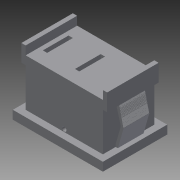
# Autodesk Inventor part: Base
Saved by Autodesk Inventor 2015 (Build 190159000, 159)
## iProperties
Created: 2016-05-14
Part Number: Base
Material: Genérico
Document SubType Name: Modeling
Designer: Isra
Density: 1 g/cm^3
Appearance: Valor por defecto
Author: Isra
Autodesk Inventor part; units mm, degrees
ref_plane "YZ Plane" through (0, 0, 0) normal (1, 0, 0) x (0, 1, 0)
ref_plane "XZ Plane" through (0, 0, 0) normal (0, 1, 0) x (-1, 0, 0)
ref_plane "XY Plane" through (0, 0, 0) normal (0, 0, 1) x (1, 0, 0)
sketch "Boceto1" plane through (0, 0, 0) normal (0, 0, 1) x (1, 0, 0)
  line L0 (10.5, -7.5) -> (-10.5, -7.5)
  line L1 (-10.5, -7.5) -> (-10.5, 7.5)
  line L2 (-10.5, 7.5) -> (10.5, 7.5)
  line L3 (10.5, 7.5) -> (10.5, -7.5)
  line L4 (10.5, -7.5) -> (-10.5, 7.5) construction
  line L5 (-10.5, -7.5) -> (10.5, 7.5) construction
  point P0 (0, 0)
  dimension "d0" = 21
  dimension "d1" = 15
  constraints: 12 end point, 2 midpoint, 2 parallel, 1 horizontal, 1 perpendicular
  measures "d0" distance of L1.end L2.end
  measures "d1" distance of L0.end L1.end
extrude "Extrusión1" add sketch "Boceto1" along normal blind 2
sketch "Boceto2" plane through (0, 0, 2) normal (0, 0, 1) x (1, 0, 0)
  line L0 (9, -6) -> (-9, -6)
  line L1 (-9, -6) -> (-9, 6)
  line L2 (-9, 6) -> (9, 6)
  line L3 (9, 6) -> (9, -6)
  line L4 (9, -6) -> (-9, 6) construction
  line L5 (-9, -6) -> (9, 6) construction
  point P0 (0, 0)
  dimension "d4" = 18
  dimension "d5" = 12
  constraints: 12 end point, 2 midpoint, 2 parallel, 1 horizontal, 1 perpendicular
  measures "d4" distance of L1.end L2.end
  measures "d5" distance of L0.end L1.end
extrude "Extrusión2" add sketch "Boceto2" along normal blind 11
sketch "Boceto3" plane through (-9, -6, 2) normal (0, -1, 0) x (1, 0, 0)
  line L0 (18, 11) -> (18, 13)
  line L1 (18, 13) -> (19, 13)
  line L2 (19, 13) -> (19, 9)
  line L3 (19, 9) -> (18, 9)
  line L4 (18, 0) -> (18, 11) projected
  line L5 (18, 9) -> (18, 11)
  point P0 (9, -2)
  dimension "d8" = 2
  dimension "d9" = 1
  dimension "d10" = 4
  dimension "d11" = 1
  constraints: 10 end point, 2 perpendicular, 1 collinear, 1 point on line, 1 vertical
  measures "d8" distance of L0.start L0.end
  measures "d9" distance of L0.end L1.end
  measures "d10" distance of L1.end L2.end
  measures "d11" distance of L2.end L3.end
extrude "Extrusión3" add sketch "Boceto3" against normal blind 12
ref_plane "Plano de trabajo1" through (0, -6, 2) normal (1, 0, 0) x (0, 0, -1)
mirror "Simetría1" about plane through (0, -6, 2) normal (1, 0, 0) of "Extrusión3"
sketch "Boceto4" plane through (0, -6, 2) normal (-1, 0, 0) x (0, 0, -1)
  point P0 (2, 6)
ref_plane "Plano de trabajo3" through (-9, 0, 2) normal (0, -1, 0) x (1, 0, 0)
sketch "Boceto5" plane through (-9, 0, 2) normal (0, -1, 0) x (1, 0, 0)
  line L0 (18, 0) -> (18, 9) projected
  line L1 (18, 9) -> (19, 9) projected
  line L2 (19, 9) -> (18, 9) projected
  line L3 (0, 0) -> (18, 0) projected
  line L4 (18, 0) -> (0, 0) projected
  line L5 (-1.5, 0) -> (19.5, 0) projected
  line L6 (19.5, 0) -> (-1.5, 0) projected
  line L7 (18.7905, 9) -> (19.8289, 4.7159)
  line L8 (19.8289, 4.7159) -> (18.5, 0)
  line L9 (-1.5, 0) -> (19.5, 0) projected
  line L10 (18.5, 0) -> (18, 0)
  line L11 (18.7905, 9) -> (18, 9)
  point P0 (9, -2)
  constraints: 8 end point, 1 collinear, 1 horizontal, 1 point on line, 2 other
extrude "Extrusión4" add sketch "Boceto5" along normal blind 3 separate body
sketch "Boceto6" plane through (-9, 0, 2) normal (0, 1, 0) x (1, 0, 0)
  line L0 (18, -9) -> (18, 0) projected
  line L1 (18, 0) -> (18, -9) projected
  line L2 (18, -0.6327) -> (19.1944, -4.78)
  line L3 (19.1944, -4.78) -> (18, -9)
  line L4 (18, -9) -> (18, -0.6327)
  point P0 (9, 2)
  constraints: 6 end point, 1 collinear, 1 point on line
extrude "Extrusión5" cut sketch "Boceto6" against normal blind 3 bodies 2
sketch "Boceto8" plane through (-9, 0, 2) normal (0, 1, 0) x (1, 0, 0)
  line L0 (19.9491, -4.6303) -> (19.748, -4.8063)
  line L1 (19.748, -4.8063) -> (19.874, -4.9502)
  line L2 (19.874, -4.9502) -> (20.0751, -4.7743)
  line L3 (20.0751, -4.7743) -> (19.9491, -4.6303)
  line L4 (19.9169, -4.752) -> (19.7158, -4.928)
  line L5 (19.7158, -4.928) -> (19.8418, -5.072)
  line L6 (19.8418, -5.072) -> (20.0429, -4.896)
  line L7 (20.0429, -4.896) -> (19.9169, -4.752)
  line L8 (19.8931, -4.857) -> (19.692, -5.033)
  line L9 (19.692, -5.033) -> (19.818, -5.1769)
  line L10 (19.818, -5.1769) -> (20.0191, -5.0009)
  line L11 (20.0191, -5.0009) -> (19.8931, -4.857)
  line L12 (19.8635, -4.9773) -> (19.6624, -5.1533)
  line L13 (19.6624, -5.1533) -> (19.7883, -5.2972)
  line L14 (19.7883, -5.2972) -> (19.9895, -5.1212)
  line L15 (19.9895, -5.1212) -> (19.8635, -4.9773)
  line L16 (19.8344, -5.0996) -> (19.6333, -5.2756)
  line L17 (19.6333, -5.2756) -> (19.7593, -5.4196)
  line L18 (19.7593, -5.4196) -> (19.9604, -5.2436)
  line L19 (19.9604, -5.2436) -> (19.8344, -5.0996)
  line L20 (19.8044, -5.2221) -> (19.6033, -5.3981)
  line L21 (19.6033, -5.3981) -> (19.7293, -5.5421)
  line L22 (19.7293, -5.5421) -> (19.9304, -5.3661)
  line L23 (19.9304, -5.3661) -> (19.8044, -5.2221)
  line L24 (19.7757, -5.3446) -> (19.5745, -5.5206)
  line L25 (19.5745, -5.5206) -> (19.7005, -5.6646)
  line L26 (19.7005, -5.6646) -> (19.9016, -5.4886)
  line L27 (19.9016, -5.4886) -> (19.7757, -5.3446)
  line L28 (19.7457, -5.4697) -> (19.5445, -5.6456)
  line L29 (19.5445, -5.6456) -> (19.6705, -5.7896)
  line L30 (19.6705, -5.7896) -> (19.8716, -5.6136)
  line L31 (19.8716, -5.6136) -> (19.7457, -5.4697)
  line L32 (19.7144, -5.5909) -> (19.5133, -5.7669)
  line L33 (19.5133, -5.7669) -> (19.6392, -5.9109)
  line L34 (19.6392, -5.9109) -> (19.8404, -5.7349)
  line L35 (19.8404, -5.7349) -> (19.7144, -5.5909)
  line L36 (19.6844, -5.7159) -> (19.4833, -5.8919)
  line L37 (19.4833, -5.8919) -> (19.6092, -6.0359)
  line L38 (19.6092, -6.0359) -> (19.8104, -5.8599)
  line L39 (19.8104, -5.8599) -> (19.6844, -5.7159)
  line L40 (19.6557, -5.8384) -> (19.4545, -6.0144)
  line L41 (19.4545, -6.0144) -> (19.5805, -6.1584)
  line L42 (19.5805, -6.1584) -> (19.7816, -5.9824)
  line L43 (19.7816, -5.9824) -> (19.6557, -5.8384)
  line L44 (19.6257, -5.9609) -> (19.4245, -6.1369)
  line L45 (19.4245, -6.1369) -> (19.5505, -6.2809)
  line L46 (19.5505, -6.2809) -> (19.7516, -6.1049)
  line L47 (19.7516, -6.1049) -> (19.6257, -5.9609)
  line L48 (19.5969, -6.0797) -> (19.3958, -6.2557)
  line L49 (19.3958, -6.2557) -> (19.5217, -6.3996)
  line L50 (19.5217, -6.3996) -> (19.7229, -6.2236)
  line L51 (19.7229, -6.2236) -> (19.5969, -6.0797)
  line L52 (19.5669, -6.1997) -> (19.3658, -6.3757)
  line L53 (19.3658, -6.3757) -> (19.4917, -6.5196)
  line L54 (19.4917, -6.5196) -> (19.6929, -6.3437)
  line L55 (19.6929, -6.3437) -> (19.5669, -6.1997)
  line L56 (19.5369, -6.3235) -> (19.3358, -6.4994)
  line L57 (19.3358, -6.4994) -> (19.4617, -6.6434)
  line L58 (19.4617, -6.6434) -> (19.6629, -6.4674)
  line L59 (19.6629, -6.4674) -> (19.5369, -6.3235)
  line L60 (19.5202, -6.4655) -> (19.3191, -6.6415)
  line L61 (19.3191, -6.6415) -> (19.4451, -6.7855)
  line L62 (19.4451, -6.7855) -> (19.6462, -6.6095)
  line L63 (19.6462, -6.6095) -> (19.5202, -6.4655)
  line L64 (19.488, -6.5873) -> (19.2869, -6.7632)
  line L65 (19.614, -6.7312) -> (19.488, -6.5873)
  line L66 (19.2869, -6.7632) -> (19.4129, -6.9072)
  line L67 (19.4129, -6.9072) -> (19.614, -6.7312)
  line L68 (19.4643, -6.6922) -> (19.2631, -6.8682)
  line L69 (19.5902, -6.8362) -> (19.4643, -6.6922)
  line L70 (19.2631, -6.8682) -> (19.3891, -7.0121)
  line L71 (19.3891, -7.0121) -> (19.5902, -6.8362)
  line L72 (19.4346, -6.8125) -> (19.2335, -6.9885)
  line L73 (19.5606, -6.9565) -> (19.4346, -6.8125)
  line L74 (19.2335, -6.9885) -> (19.3594, -7.1324)
  line L75 (19.3594, -7.1324) -> (19.5606, -6.9565)
  line L76 (19.4055, -6.9349) -> (19.2044, -7.1109)
  line L77 (19.5315, -7.0788) -> (19.4055, -6.9349)
  line L78 (19.2044, -7.1109) -> (19.3304, -7.2548)
  line L79 (19.3304, -7.2548) -> (19.5315, -7.0788)
  line L80 (19.3755, -7.0574) -> (19.1744, -7.2334)
  line L81 (19.5015, -7.2013) -> (19.3755, -7.0574)
  line L82 (19.1744, -7.2334) -> (19.3004, -7.3773)
  line L83 (19.3004, -7.3773) -> (19.5015, -7.2013)
  line L84 (19.3468, -7.1799) -> (19.1457, -7.3559)
  line L85 (19.4727, -7.3238) -> (19.3468, -7.1799)
  line L86 (19.1457, -7.3559) -> (19.2716, -7.4998)
  line L87 (19.2716, -7.4998) -> (19.4727, -7.3238)
  line L88 (19.3168, -7.3049) -> (19.1156, -7.4809)
  line L89 (19.4427, -7.4488) -> (19.3168, -7.3049)
  line L90 (19.1156, -7.4809) -> (19.2416, -7.6248)
  line L91 (19.2416, -7.6248) -> (19.4427, -7.4488)
  line L92 (19.2855, -7.4262) -> (19.0844, -7.6021)
  line L93 (19.4115, -7.5701) -> (19.2855, -7.4262)
  line L94 (19.0844, -7.6021) -> (19.2104, -7.7461)
  line L95 (19.2104, -7.7461) -> (19.4115, -7.5701)
  line L96 (19.2555, -7.5512) -> (19.0544, -7.7271)
  line L97 (19.3815, -7.6951) -> (19.2555, -7.5512)
  line L98 (19.0544, -7.7271) -> (19.1804, -7.8711)
  line L99 (19.1804, -7.8711) -> (19.3815, -7.6951)
  line L100 (19.2268, -7.6737) -> (19.0256, -7.8497)
  line L101 (19.3527, -7.8176) -> (19.2268, -7.6737)
  line L102 (19.0256, -7.8497) -> (19.1516, -7.9936)
  line L103 (19.1516, -7.9936) -> (19.3527, -7.8176)
  line L104 (19.1968, -7.7962) -> (18.9956, -7.9722)
  line L105 (19.3227, -7.9401) -> (19.1968, -7.7962)
  line L106 (18.9956, -7.9722) -> (19.1216, -8.1161)
  line L107 (19.1216, -8.1161) -> (19.3227, -7.9401)
  line L108 (19.168, -7.9149) -> (18.9669, -8.0909)
  line L109 (19.294, -8.0589) -> (19.168, -7.9149)
  line L110 (18.9669, -8.0909) -> (19.0928, -8.2349)
  line L111 (19.0928, -8.2349) -> (19.294, -8.0589)
  line L112 (19.138, -8.0349) -> (18.9369, -8.2109)
  line L113 (19.264, -8.1789) -> (19.138, -8.0349)
  line L114 (18.9369, -8.2109) -> (19.0628, -8.3549)
  line L115 (19.0628, -8.3549) -> (19.264, -8.1789)
  line L116 (19.108, -8.1587) -> (18.9069, -8.3347)
  line L117 (19.234, -8.3027) -> (19.108, -8.1587)
  line L118 (18.9069, -8.3347) -> (19.0328, -8.4786)
  line L119 (19.0328, -8.4786) -> (19.234, -8.3027)
  line L120 (19.2164, -8.3959) -> (19.0904, -8.2519)
  line L121 (19.0904, -8.2519) -> (18.8893, -8.4279)
  line L122 (19.0153, -8.5719) -> (19.2164, -8.3959)
  line L123 (18.8893, -8.4279) -> (19.0153, -8.5719)
  line L124 (19.1846, -8.495) -> (19.0586, -8.3511)
  line L125 (19.0586, -8.3511) -> (18.8575, -8.5271)
  line L126 (18.9835, -8.671) -> (19.1846, -8.495)
  line L127 (18.8575, -8.5271) -> (18.9835, -8.671)
  line L128 (19.1595, -8.5942) -> (19.0335, -8.4503)
  line L129 (19.0335, -8.4503) -> (18.8324, -8.6262)
  line L130 (18.9583, -8.7702) -> (19.1595, -8.5942)
  line L131 (18.8324, -8.6262) -> (18.9583, -8.7702)
  line L132 (19.1343, -8.6934) -> (19.0084, -8.5494)
  line L133 (19.0084, -8.5494) -> (18.8072, -8.7254)
  line L134 (18.9332, -8.8694) -> (19.1343, -8.6934)
  line L135 (18.8072, -8.7254) -> (18.9332, -8.8694)
  line L136 (19.1078, -8.8003) -> (18.9818, -8.6563)
  line L137 (18.9818, -8.6563) -> (18.7807, -8.8323)
  line L138 (18.9067, -8.9763) -> (19.1078, -8.8003)
  line L139 (18.7807, -8.8323) -> (18.9067, -8.9763)
  line L140 (18.9067, -8.9763) -> (18.7653, -8.942)
  line L141 (19.8289, -4.7159) -> (18.7905, -9) projected
  line L142 (18.7653, -8.942) -> (18.8202, -8.8775)
  point P0 (9, 2)
  constraints: 284 end point, 71 perpendicular, 35 parallel, 2 point on line
extrude "Extrusión6" cut sketch "Boceto8" against normal blind 3 contours L3 L2 L7 L4 L141 L0 | L141 L1 L0 | L4 L7 L2 L11 L8 L1 | L141 L8 L5 L4 | L1 L8 L141 | L7 L6 L11 L2 | L8 L11 L2 L1 | L1 L2 L11 L6 L15 L12 L5 L141 L8 | L141 L5 L8 | L5 L141 L9 L8 | L5 L12 L141 | L11 L10 L15 L6 | L12 L15 L6 L5 | L5 L6 L15 L10 L19 L16 L9 L12 | L141 L13 L12 | L9 L16 L141 | L16 L19 L10 L9 | L9 L10 L19 L14 L23 L20 L13 L16 | L141 L17 L16 | L13 L20 L141 | L15 L14 L19 L10 | L20 L23 L14 L13 | L13 L14 L23 L18 L27 L24 L17 L20 | L141 L21 L20 | L17 L24 L141 | L24 L27 L18 L17 | L17 L18 L27 L22 L31 L28 L21 L24 | L141 L25 L24 | L21 L28 L141 | L19 L18 L23 L14 | L28 L31 L22 L21 | L21 L22 L31 L26 L35 L32 L25 L28 | L141 L29 L28 | L25 L32 L141 | L23 L22 L27 L18 | L32 L35 L26 L25 | L25 L26 L35 L30 L39 L36 L29 L32 | L141 L33 L32 | L29 L36 L141 | L27 L26 L31 L22 | L36 L39 L30 L29 | L29 L30 L39 L34 L43 L40 L33 L36 | L141 L37 L36 | L33 L40 L141 | L31 L30 L35 L26 | L40 L43 L34 L33 | L33 L34 L43 L38 L47 L44 L37 L40 | L141 L41 L40 | L37 L44 L141 | L35 L34 L39 L30 | L44 L47 L38 L37 | L37 L38 L47 L42 L51 L48 L41 L44 | L141 L45 L44 | L41 L48 L141 | L39 L38 L43 L34 | L48 L51 L42 L41 | L41 L42 L51 L46 L55 L52 L45 L48 | L141 L49 L48 | L45 L52 L141 | L43 L42 L47 L38 | L52 L55 L46 L45 | L45 L46 L55 L50 L59 L56 L49 L52 | L141 L53 L52 | L49 L56 L141 | L47 L46 L51 L42 | L56 L59 L50 L49 | L49 L50 L59 L54 L63 L60 L53 L56 | L141 L57 L56 | L53 L60 L57 L141 | L51 L50 L55 L46 | L60 L63 L54 L53 | L53 L54 L63 L58 L65 L64 L57 L60 | L55 L54 L59 L50 | L57 L64 L61 L141 L60 | L141 L61 L60 | L59 L58 L63 L54 | L64 L65 L58 L57 | L57 L58 L65 L62 L69 L68 L61 L64 | L63 L62 L65 L58 | L61 L68 L66 L141 L64 | L141 L66 L64 | L68 L69 L62 L61 | L61 L62 L69 L67 L73 L72 L66 L68 | L65 L67 L69 L62 | L66 L72 L70 L141 L68 | L141 L70 L68 | L72 L73 L67 L66 | L66 L67 L73 L71 L77 L76 L70 L72 | L69 L71 L73 L67 | L70 L76 L74 L141 L72 | L141 L74 L72 | L76 L77 L71 L70 | L70 L71 L77 L75 L81 L80 L74 L76 | L73 L75 L77 L71 | L74 L80 L78 L141 L76 | L141 L78 L76 | L80 L81 L75 L74 | L74 L75 L81 L79 L85 L84 L78 L80 | L77 L79 L81 L75 | L78 L84 L82 L141 L80 | L141 L82 L80 | L84 L85 L79 L78 | L78 L79 L85 L83 L89 L88 L82 L84 | L81 L83 L85 L79 | L82 L88 L86 L141 L84 | L141 L86 L84 | L88 L89 L83 L82 | L82 L83 L89 L87 L93 L92 L86 L88 | L85 L87 L89 L83 | L86 L92 L90 L141 L88 | L141 L90 L88 | L92 L93 L87 L86 | L86 L87 L93 L91 L97 L96 L90 L92 | L89 L91 L93 L87 | L90 L96 L94 L141 L92 | L141 L94 L92 | L96 L97 L91 L90 | L90 L91 L97 L95 L101 L100 L94 L96 | L93 L95 L97 L91 | L94 L100 L98 L141 L96 | L141 L98 L96 | L100 L101 L95 L94 | L94 L95 L101 L99 L105 L104 L98 L100 | L97 L99 L101 L95 | L98 L104 L102 L141 L100 | L141 L102 L100 | L104 L105 L99 L98 | L98 L99 L105 L103 L109 L108 L102 L104 | L101 L103 L105 L99 | L102 L108 L106 L141 L104 | L141 L106 L104 | L108 L109 L103 L102 | L102 L103 L109 L107 L113 L112 L106 L108 | L105 L107 L109 L103 | L106 L112 L110 L141 L108 | L141 L110 L108 | L112 L113 L107 L106 | L106 L107 L113 L111 L117 L116 L110 L112 | L109 L111 L113 L107 | L110 L116 L114 L141 L112 | L141 L114 L112 | L116 L117 L111 L110 | L110 L111 L117 L115 L120 L121 L114 L116 | L113 L115 L117 L111 | L114 L121 L118 L141 L116 | L141 L118 L116 | L121 L120 L115 L114 | L114 L125 L118 L121 | L117 L119 L120 L115 | L114 L124 L119 L128 L129 L118 L125 | L118 L125 L123 L141 L121 | L141 L123 L121 | L120 L119 L124 L115 | L118 L129 L123 L125 | L120 L122 L124 L119 | L124 L122 L128 L119 | L129 L128 L119 L118 | L118 L119 L128 L122 L132 L133 L123 L129 | L123 L129 L141 L125 | L141 L127 L125 | L124 L126 L128 L122 | L123 L133 L127 L129 | L141 L131 L129 | L127 L133 L141 | L128 L126 L132 L122 | L133 L132 L122 L123 | L123 L122 L132 L126 L136 L137 L127 L133 | L127 L137 L131 L133 | L141 L135 L133 | L131 L137 L141 | L128 L130 L132 L126 | L137 L136 L126 L127 | L127 L126 L136 L130 L131 L137 | L131 L130 L136 L134 L135 L137 | L141 L139 L137 | L135 L134 L136 L138 L139 L141 | L132 L130 L136 L126 | L139 L140 L141 | L141 L140 L142 | L132 L134 L136 L130 bodies 2
ref_plane "Plano de trabajo4" through (0, -6, 2) normal (1, 0, 0) x (0, 0, -1)
mirror "Simetría2" about plane through (0, -6, 2) normal (1, 0, 0) bodies 2
sketch "Boceto9" plane through (0, 0, 0) normal (0, 0, -1) x (-1, 0, 0)
  line L0 (8, 5) -> (-8, 5)
  line L1 (-8, 5) -> (-8, -5)
  line L2 (-8, -5) -> (8, -5)
  line L3 (8, -5) -> (8, 5)
  line L4 (8, 5) -> (-8, -5) construction
  line L5 (-8, 5) -> (8, -5) construction
  point P0 (0, 0)
  dimension "d20" = 16
  dimension "d21" = 10
  constraints: 12 end point, 2 midpoint, 2 parallel, 1 horizontal, 1 perpendicular
  measures "d20" distance of L2.end L1.end
  measures "d21" distance of L1.end L0.end
extrude "Extrusión7" cut sketch "Boceto9" against normal blind 12 bodies 1
hole "Agujero1" at (0, 6, 2.6) direction (0, -1, 0) diameter 1 end through all bodies 1
mirror "Simetría3" about plane through (-9, 0, 2) normal (0, -1, 0) bodies 2
sketch "Boceto10" plane through (0, 0, 13) normal (0, 0, 1) x (1, 0, 0)
  line L0 (-9, -6) -> (-9, 6) projected
  line L1 (9, -6) -> (9, 6) projected
  line L2 (0.5, -3) -> (-0.5, -3)
  line L3 (-0.5, -3) -> (-0.5, 3)
  line L4 (-0.5, 3) -> (0.5, 3)
  line L5 (0.5, 3) -> (0.5, -3)
  line L6 (0.5, -3) -> (-0.5, 3) construction
  line L7 (-0.5, -3) -> (0.5, 3) construction
  line L8 (8, -3) -> (7, -3)
  line L9 (7, -3) -> (7, 3)
  line L10 (7, 3) -> (8, 3)
  line L11 (8, 3) -> (8, -3)
  line L12 (-7, -3) -> (-8, -3)
  line L13 (-8, -3) -> (-8, 3)
  line L14 (-8, 3) -> (-7, 3)
  line L15 (-7, 3) -> (-7, -3)
  point P0 (0, 0)
  dimension "d33" = 1
  dimension "d34" = 6
  dimension "d35" = 1
  dimension "d36" = 6
  dimension "d37" = 1
  dimension "d38" = 6
  dimension "d39" = 1
  dimension "d40" = 1
  constraints: 28 end point, 6 parallel, 3 horizontal, 3 perpendicular, 2 midpoint
  measures "d33" distance of L3.end L4.end
  measures "d34" distance of L2.end L3.end
  measures "d35" distance of L9.end L11.start
  measures "d36" distance of L9.start L9.end
  measures "d37" distance of L13.end L15.start
  measures "d38" distance of L13.start L13.end
  measures "d39" distance between parallel lines of L13 L0
  measures "d40" distance between parallel lines of L1 L11
extrude "Extrusión8" cut sketch "Boceto10" against normal blind 2 bodies 1
ref_plane "Plano de trabajo2" through (0, -6, 2) normal (1, 0, 0) x (0, 0, -1)
